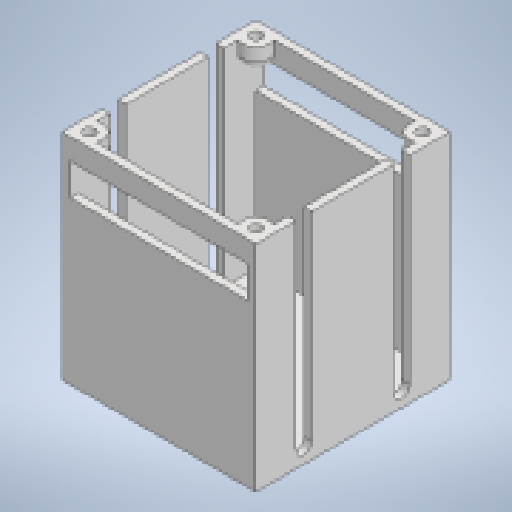
# Autodesk Inventor part: Base dispensador
Saved by Autodesk Inventor 2024 (Build 280153000, 153)
## iProperties
Created: 2025-03-02
Part Number: Base dispensador
Material: Genérico
Document SubType Name: Modeling
Designer: sergi
Density: 1 g/cm^3
Appearance: Valor por defecto
Author: sergi
Autodesk Inventor part; units mm, degrees
ref_plane "YZ Plane" through (0, 0, 0) normal (1, 0, 0) x (0, 1, 0)
ref_plane "XZ Plane" through (0, 0, 0) normal (0, 1, 0) x (-1, 0, 0)
ref_plane "XY Plane" through (0, 0, 0) normal (0, 0, 1) x (1, 0, 0)
ref_plane "Plano de trabajo2" through (-39.5, 85, -114.5) normal (0, 1, 0) x (0, 0, 1)
sketch "Boceto1" plane through (0, 0, 0) normal (0, 1, 0) x (-1, 0, 0)
  line L0 (-36.5, -36.5) -> (36.5, -36.5)
  line L1 (36.5, -36.5) -> (36.5, 36.5)
  line L2 (36.5, 36.5) -> (-36.5, 36.5)
  line L3 (-36.5, 36.5) -> (-36.5, -36.5)
  line L4 (-36.5, -36.5) -> (36.5, 36.5) construction
  line L5 (36.5, -36.5) -> (-36.5, 36.5) construction
  point P0 (0, 0)
  dimension "d0" = 73
  dimension "d1" = 73
  constraints: 12 end point, 2 midpoint, 2 parallel, 1 horizontal, 1 perpendicular
  measures "d0" distance of L2.end L1.end
  measures "d1" distance of L1.end L0.end
extrude "Extrusión1" add sketch "Boceto1" along normal blind 81
ref_plane "Plano de trabajo1" through (-39.5, 85, -114.5) normal (0, 1, 0) x (0, 0, 1)
sketch "Boceto4" plane through (0, 81, 0) normal (0, 1, 0) x (1, 0, 0)
  line L0 (-36.5, 36.5) -> (-36.5, -36.5) projected
  line L1 (-36.5, -36.5) -> (36.5, -36.5) projected
  line L2 (36.5, -36.5) -> (36.5, 36.5) projected
  line L3 (36.5, 36.5) -> (-36.5, 36.5) projected
  line L4 (-33.5, -33.5) -> (-33.5, 33.5)
  line L5 (-33.5, 33.5) -> (33.5, 33.5)
  line L6 (33.5, 33.5) -> (33.5, -33.5)
  line L7 (33.5, -33.5) -> (-33.5, -33.5)
  circle A0 centre (-31.4, 31.4) radius 2.1
  circle A1 centre (-31.4, -31.4) radius 2.1
  circle A2 centre (31.4, -31.4) radius 2.1
  circle A3 centre (31.4, 31.4) radius 2.1
  point P0 (0, 0)
  dimension "d22" = 3
  dimension "d23" = 4.2
  dimension "d26" = 360
  constraints: 8 end point, 4 centre point, 2 tangent, 12 other
  measures "d22" distance between parallel lines of L0 L4
  measures "d23" diameter of A0
hole "Agujero2" at (-31.4, 81, -31.4) at (-31.4, 81, 31.4) at (31.4, 81, 31.4) at (31.4, 81, -31.4) direction (0, -1, 0) diameter 4.2 depth 5
shell "Vaciado2" thickness 3 removed faces 1 at (-10.0025, 81, -9.9427)
fillet "Empalme2" radius 3 4 edges at (-27.7938, 73, -27.7938) (27.7938, 73, -27.7938) (27.7938, 73, 27.7938) (-27.7938, 73, 27.7938)
sketch "Boceto5" plane through (36.5, 0, 36.5) normal (1, 0, 0) x (0, 0, -1)
  line L0 (0, 0) -> (73, 0) projected
  line L1 (73, 0) -> (73, 81) projected
  line L2 (0, 81) -> (73, 81) projected
  line L3 (0, 0) -> (0, 81) projected
  line L4 (63.2524, 81) -> (63.2524, 76) projected
  line L5 (9.7476, 76) -> (9.7476, 81) projected
  line L6 (10.2, 76) -> (10.2, 81) projected
  line L7 (62.8, 76) -> (62.8, 81) projected
  line L8 (15, 66) -> (58, 66)
  line L9 (58, 81) -> (58, 0)
  line L10 (58, 15) -> (15, 15)
  line L11 (15, 0) -> (15, 81)
  line L12 (21, 0) -> (21, 81)
  line L13 (52, 81) -> (52, 0)
  line L14 (70, 3) -> (3, 3)
  line L15 (3, 3) -> (3, 78)
  line L16 (3, 78) -> (70, 78)
  line L17 (70, 78) -> (70, 3)
  point P0 (36.5, 0)
  point P1 (52, 3)
  point P2 (58, 3)
  point P3 (58, 78)
  point P4 (52, 78)
  point P5 (21, 78)
  point P6 (15, 78)
  point P7 (15, 3)
  point P8 (21, 3)
  point P9 (52, 81)
  point P10 (21, 81)
  dimension "d37" = 15
  dimension "d38" = 6
  dimension "d39" = 6
  dimension "d40" = 3
  constraints: 20 end point, 8 point on line, 2 parallel, 3 other
  measures "d37" distance between parallel lines of L3 L11
  measures "d38" distance between parallel lines of L11 L12
  measures "d39" distance between parallel lines of L9 L13
  measures "d40" distance between parallel lines of L0 L14
extrude "Extrusión3" cut sketch "Boceto5" against normal through all contours L11 L10 L12 L14 | L11 L8 L12 L10 | L13 L10 L9 L14 | L11 L16 L12 L8 | L2 L12 L16 L11 | L13 L8 L9 L10 | L13 L16 L9 L8 | L2 L9 L16 L13
fillet "Empalme3" radius 3 8 edges at (-35, 3, -21.5) (-35, 3, -15.5) (-35, 3, 15.5) (-35, 3, 21.5) (35, 3, 15.5) (35, 3, 21.5) (35, 3, -21.5) (35, 3, -15.5)
sketch "Boceto6" plane through (36.5, 0, -36.5) normal (0, 0, -1) x (-1, 0, 0)
  line L0 (0, 0) -> (73, 0) projected
  line L1 (73, 0) -> (73, 81) projected
  line L2 (0, 81) -> (73, 81) projected
  line L3 (0, 0) -> (0, 81) projected
  line L4 (67.9, 73) -> (70, 73) projected
  line L5 (3, 73) -> (5.1, 73) projected
  line L6 (3, 78) -> (70, 78)
  line L7 (70, 78) -> (70, 3)
  line L8 (70, 3) -> (3, 3)
  line L9 (3, 3) -> (3, 78)
  line L10 (3, 73) -> (70, 73)
  line L11 (70, 73) -> (70, 61)
  line L12 (70, 61) -> (3, 61)
  line L13 (3, 61) -> (3, 73)
  point P0 (36.5, 0)
  point P1 (3, 61)
  point P2 (3, 73)
  dimension "d44" = 12
  constraints: 16 end point, 2 parallel, 1 horizontal, 1 perpendicular, 1 point on line, 5 other
  measures "d44" distance of L10.end L11.end
extrude "Extrusión4" cut sketch "Boceto6" against normal through all contours L4 L7 L12 L9 L5 L10
